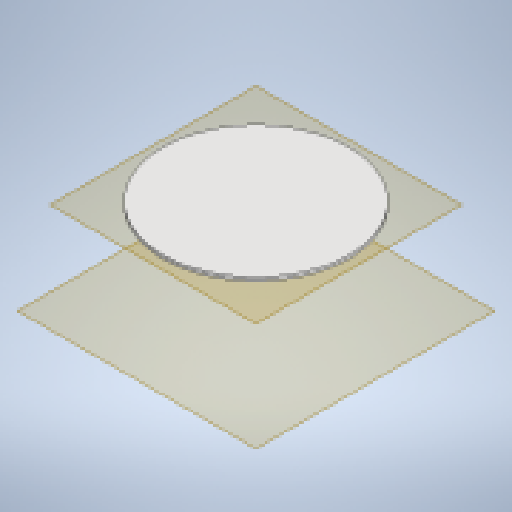
# Autodesk Inventor part: Deckel
Saved by Autodesk Inventor 2024 (Build 280153000, 153)
## iProperties
Created: 2024-01-25
Part Number: Deckel
Material: Generic
Document SubType Name: Modeling
Designer: Daniel Nussbaum
Density: 1 g/cm^3
Appearance: Default
Author: Daniel Nussbaum
Autodesk Inventor part; units mm, degrees
ref_plane "YZ Plane" through (0, 0, 0) normal (1, 0, 0) x (0, 1, 0)
ref_plane "XZ Plane" through (0, 0, 0) normal (0, 1, 0) x (-1, 0, 0)
ref_plane "XY Plane" through (0, 0, 0) normal (0, 0, 1) x (1, 0, 0)
sketch "Sketch2" plane through (0, 0, 0) normal (0, 1, 0) x (-1, 0, 0)
  arc A0 (-485.8905, 731.6468) -> (-682.1657, 423.2838) centre (-406.1929, 464.272) ccw projected
  circle A1 centre (-406.1929, 464.272) radius 279
  circle A2 centre (-406.1929, 464.272) radius 278
  point P0 (0, 0)
  dimension "d4" = 1
  constraints: 2 centre point, 1 coincident, 1 concentric
  measures "d4" radial gap between concentric circles of A1 A2
extrude "Extrusion2" add sketch "Sketch2" along normal blind 10 contours A2
body "Solid2"
